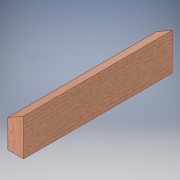
# Autodesk Inventor part: BA06
Saved by Autodesk Inventor 2017 (Build 210142000, 142)
## iProperties
Created: 2018-10-18
Part Number: BA06
Material: Wood (Oak)
Document SubType Name: Modeling
Designer: Dell
Density: 0.76 g/cm^3
Appearance: White Oak - Natural Medium Gloss
Author: Dell
Autodesk Inventor part; units mm, degrees
ref_plane "YZ Plane" through (0, 0, 0) normal (1, 0, 0) x (0, 1, 0)
ref_plane "XZ Plane" through (0, 0, 0) normal (0, 1, 0) x (-1, 0, 0)
ref_plane "XY Plane" through (0, 0, 0) normal (0, 0, 1) x (1, 0, 0)
sketch "Sketch1" plane through (0, 0, 0) normal (0, 0, 1) x (1, 0, 0)
  line L0 (0, 0) -> (38.1, 0)
  line L1 (38.1, 0) -> (38.1, 88.9)
  line L2 (38.1, 88.9) -> (0, 88.9)
  line L3 (0, 88.9) -> (0, 0)
  dimension "d0" = 38.1
  dimension "d1" = 88.9
  constraints: 8 end point, 2 parallel, 1 horizontal, 1 perpendicular
  measures "d0" distance of L2.end L1.end
  measures "d1" distance of L1.end L0.end
extrude "Extrusion1" add sketch "Sketch1" along normal blind 355.6
sketch "Sketch2" plane through (0, 0, 355.6) normal (0, 0, 1) x (1, 0, 0)
  line L0 (38.1, 0) -> (38.1, 88.9) projected
  line L1 (38.1, 88.9) -> (0, 66.903)
  line L2 (0, 88.9) -> (0, 0) projected
  line L3 (0, 66.903) -> (0, 88.9)
  line L4 (0, 88.9) -> (38.1, 88.9)
  dimension "d4" = 30
  constraints: 6 end point, 1 collinear, 1 perpendicular
  measures "d4" angle of L4 L1
extrude "Extrusion2" cut sketch "Sketch2" against normal through all
body "Solid1"
